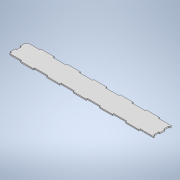
# Autodesk Inventor part: base
Saved by Autodesk Inventor 2020 (Build 240168000, 168)
## iProperties
Created: 2020-03-06
Part Number: base
Material: Generic
Document SubType Name: Modeling
Designer: udvarhelyi
Density: 1 g/cm^3
Appearance: Default
Author: udvarhelyi
Autodesk Inventor part; units mm, degrees
ref_plane "YZ Plane" through (0, 0, 0) normal (1, 0, 0) x (0, 1, 0)
ref_plane "XZ Plane" through (0, 0, 0) normal (0, 1, 0) x (-1, 0, 0)
ref_plane "XY Plane" through (0, 0, 0) normal (0, 0, 1) x (1, 0, 0)
sketch "Sketch1" plane through (0, 0, 0) normal (0, 1, 0) x (-1, 0, 0)
  line L0 (146.1818, 19) -> (146.1818, 22)
  line L1 (114.3636, 22) -> (114.3636, 19)
  line L2 (82.5455, 19) -> (82.5455, 22)
  line L3 (50.7273, 22) -> (50.7273, 19)
  line L4 (18.9091, 19) -> (18.9091, 22)
  line L5 (-12.9091, 22) -> (-12.9091, 19)
  line L6 (-44.7273, 19) -> (-44.7273, 22)
  line L7 (-76.5455, 22) -> (-76.5455, 19)
  line L8 (-108.3636, 19) -> (-108.3636, 22)
  line L9 (-140.1818, 22) -> (-140.1818, 19)
  line L10 (-172, 15) -> (-169, 15)
  line L11 (-169, 3) -> (-172, 3)
  line L12 (-169, -9) -> (-172, -9)
  line L13 (-172, -21) -> (-169, -21)
  line L14 (-140.1818, -25) -> (-140.1818, -28)
  line L15 (-108.3636, -28) -> (-108.3636, -25)
  line L16 (-76.5455, -25) -> (-76.5455, -28)
  line L17 (-44.7273, -28) -> (-44.7273, -25)
  line L18 (-12.9091, -28) -> (-12.9091, -25)
  line L19 (18.9091, -25) -> (18.9091, -28)
  line L20 (146.1818, -28) -> (146.1818, -25)
  line L21 (114.3636, -25) -> (114.3636, -28)
  line L22 (82.5455, -28) -> (82.5455, -25)
  line L23 (50.7273, -25) -> (50.7273, -28)
  line L24 (178, -21) -> (175, -21)
  line L25 (175, 15) -> (178, 15)
  line L26 (178, 3) -> (175, 3)
  line L27 (114.3636, -28) -> (146.1818, -28)
  line L28 (50.7273, -28) -> (82.5455, -28)
  line L29 (-12.9091, -28) -> (18.9091, -28)
  line L30 (178, -21) -> (178, -17)
  line L31 (178, 3) -> (178, 7)
  line L32 (178, 11) -> (178, 15)
  line L33 (146.1818, 22) -> (114.3636, 22)
  line L34 (82.5455, 22) -> (50.7273, 22)
  line L35 (18.9091, 22) -> (-12.9091, 22)
  line L36 (-44.7273, 22) -> (-76.5455, 22)
  line L37 (-108.3636, 22) -> (-140.1818, 22)
  line L38 (-169, 15) -> (-169, 11)
  line L39 (-169, 7) -> (-169, 3)
  line L40 (-172, 3) -> (-172, -1)
  line L41 (-172, 19) -> (-172, 15)
  line L42 (-140.1818, -28) -> (-108.3636, -28)
  line L43 (-76.5455, -28) -> (-44.7273, -28)
  line L44 (-169, -9) -> (-169, -13)
  line L45 (-169, -17) -> (-169, -21)
  line L46 (-172, -5) -> (-172, -9)
  line L47 (-172, -21) -> (-172, -25)
  line L48 (-172, -25) -> (-140.1818, -25)
  line L49 (-108.3636, -25) -> (-76.5455, -25)
  line L50 (-44.7273, -25) -> (-12.9091, -25)
  line L51 (18.9091, -25) -> (50.7273, -25)
  line L52 (82.5455, -25) -> (114.3636, -25)
  line L53 (146.1818, -25) -> (175, -25)
  line L54 (175, -25) -> (175, -21)
  line L55 (175, -1) -> (175, 3)
  line L56 (175, 15) -> (175, 19)
  line L57 (175, 19) -> (146.1818, 19)
  line L58 (114.3636, 19) -> (82.5455, 19)
  line L59 (50.7273, 19) -> (18.9091, 19)
  line L60 (-12.9091, 19) -> (-44.7273, 19)
  line L61 (-76.5455, 19) -> (-108.3636, 19)
  line L62 (-140.1818, 19) -> (-172, 19)
  line L63 (178, -13) -> (178, -9)
  line L64 (178, -9) -> (175, -9)
  line L65 (175, -9) -> (175, -5)
  line L66 (-169, -17) -> (-169, -13)
  line L67 (-172, -5) -> (-172, -1)
  line L68 (-169, 7) -> (-169, 11)
  line L69 (178, -17) -> (178, -13)
  line L70 (175, -5) -> (175, -1)
  line L71 (178, 7) -> (178, 11)
  point P0 (0, 0)
  point P1 (-219, 16.6364)
  point P2 (-222, -22.6364)
  point P3 (228, -22.6364)
  dimension "d1" = 347
  dimension "d3" = 44
  dimension "d5" = 25
  dimension "d6" = 175
  dimension "d9" = 3
  dimension "d15" = 3
  dimension "d16" = 3
  dimension "d17" = 3
  dimension "d18" = 12
  dimension "d19" = 12
  dimension "d20" = 12
  dimension "d21" = 4
  dimension "d23" = 31.8182
  constraints: 167 perpendicular, 144 end point, 89 parallel, 44 collinear, 13 equal length, 6 horizontal, 3 vertical
  measures "d1" distance of L47.end L53.end
  measures "d3" distance of L53.end L56.end
  measures "d5" vertical distance of L53.end point (0, 0)
  measures "d6" horizontal distance of L53.end point (0, 0)
  measures "d9" distance of L13.start L13.end
  measures "d15" distance of L20.start L20.end
  measures "d16" distance of L0.start L0.end
  measures "d17" distance of L24.start L24.end
  measures "d18" distance between parallel lines of L64 L24
  measures "d19" distance between parallel lines of L26 L64
  measures "d20" distance between parallel lines of L25 L26
  measures "d21" distance of L53.end L24.end
  measures "d23" distance of L23.end L22.start
extrude "Extrusion1" add sketch "Sketch1" along normal blind 3
equation "\"d1\" = wt - tt"
equation "\"d3\" = -2 * tt + ht"
equation "\"d5\" = 0.5 * ht"
equation "\"d6\" = 0.5 * wt"
equation "\"d9\" = tt"
equation "\"d15\" = tt"
equation "\"d16\" = tt"
equation "\"d17\" = tt"
equation "\"d18\" = 0.272727 * ht - 0.545455 * tt"
equation "\"d19\" = d18"
equation "\"d20\" = d18"
equation "\"d21\" = -0.181818 * tt + 0.0909091 * ht"
equation "\"d23\" = 0.0909091 * wt"
equation "\"d13\" = tt"
equation "\"wt\" = 350"
equation "\"tt\" = 3"
equation "\"tol\" = 0"
equation "\"tiroir\" = 25.4"
equation "\"nHoles\" = 101.6"
equation "\"shelfH\" = 35"
equation "\"d0\" = 0.5 * wt"
equation "\"d2\" = 0.5 * lt"
equation "\"d4\" = tt"
equation "\"ht\" = 50"
equation "\"lt\" = 350"
body "Solid1"
